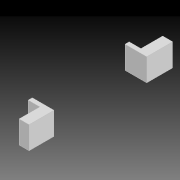
# Autodesk Inventor part: KB33-046-010 - Панель управления
Saved by Autodesk Inventor 2020 (Build 240168000, 168)
## iProperties
Created: 2021-08-16
Part Number: KB33-046-010 - Панель управления
Material: Типовые
Document SubType Name: Modeling
Designer: Петров Иван
Density: 1 g/cm^3
Appearance: По умолчанию
Mass: 31.7492 g
Surface Area: 96.0165 cm^2
Volume: 31.7492 cm^3
Author: Петров Иван
Autodesk Inventor part; units mm, degrees
ref_plane "YZ Plane" through (0, 0, 0) normal (1, 0, 0) x (0, 1, 0)
ref_plane "XZ Plane" through (0, 0, 0) normal (0, 1, 0) x (-1, 0, 0)
ref_plane "XY Plane" through (0, 0, 0) normal (0, 0, 1) x (1, 0, 0)
sketch "Эскиз1" plane through (0, 0, 0) normal (0, 1, 0) x (-1, 0, 0)
  line L0 (44.4709, 73.3307) -> (60, 73.3307)
  line L1 (44.4709, 73.3307) -> (44.4709, 28.3307)
  line L2 (44.4709, 207.0004) -> (60, 207.0004)
  line L3 (44.4709, 207.0004) -> (44.4709, 252.0004)
  line L4 (31.29, 29.5004) -> (31.29, 249.5004)
  line L5 (31.29, 201.5002) -> (60, 201.5002)
  line L6 (60, 78.8309) -> (31.29, 78.8309)
  line L7 (44.4709, 234.5004) -> (31.29, 234.5004)
  line L8 (44.4709, 44.5004) -> (31.29, 44.5004)
  line L9 (31.29, 139.5004) -> (37.8804, 139.5004)
  line L10 (60, 207.0004) -> (60, 201.5002)
  line L11 (60, 78.8309) -> (60, 73.3307)
  point P0 (0, 0)
  dimension "d0" = 5.5002
  dimension "d1" = 5.5002
  dimension "d2" = 95
  constraints: 24 end point, 5 point on line, 4 horizontal, 4 perpendicular, 3 vertical, 1 collinear, 1 midpoint, 1 other
  measures "d0" distance between parallel lines of L2 L5
  measures "d1" distance between parallel lines of L0 L6
  measures "d2" distance between parallel lines of L7 L9
extrude "Выдавливание1" add sketch "Эскиз1" along normal blind 30
equation "\"d1\" = d0"
